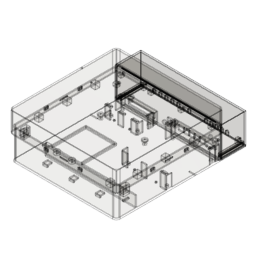
completed (Autodesk Fusion 360 design; units mm, degrees)
part number: 2026-08-16-23-06-11-456
Autodesk Fusion 360 part; units mm, degrees
(part 1 of 2)
sketch "Sketch1" plane through (0, 0, 0) normal (0, 0, 1) x (1, 0, 0)
  line L0 (140, 137) -> (-140, 137)
  line L1 (-140, 137) -> (-140, -140)
  line L2 (-140, -140) -> (140, -140)
  line L3 (140, -140) -> (140, 137)
extrude "Extrude1" add sketch "Sketch1" along normal blind 3 makes body 1
sketch "Sketch2" plane through (0, 0, 0) normal (0, 0, 1) x (1, 0, 0)
  line L0 (-137, 137) -> (-140, 137)
  line L1 (-140, 137) -> (-140, -140)
  line L2 (-140, -140) -> (-137, -140)
  line L3 (-137, -140) -> (-137, 137)
extrude "Extrude2" add sketch "Sketch2" along normal blind 77 from surface at 3 bodies 1
sketch "Sketch3" plane through (0, 0, 0) normal (0, 0, 1) x (1, 0, 0)
  line L0 (140, 137) -> (137, 137)
  line L1 (137, 137) -> (137, -140)
  line L2 (137, -140) -> (140, -140)
  line L3 (140, -140) -> (140, 137)
extrude "Extrude3" add sketch "Sketch3" along normal blind 77 from surface at 3 bodies 1
sketch "Sketch4" plane through (0, 0, 0) normal (0, 0, 1) x (1, 0, 0)
  line L0 (140, -137) -> (-140, -137)
  line L1 (-140, -137) -> (-140, -140)
  line L2 (-140, -140) -> (140, -140)
  line L3 (140, -140) -> (140, -137)
extrude "Extrude4" add sketch "Sketch4" along normal blind 77 from surface at 3 bodies 1
sketch "Sketch5" plane through (0, 0, 0) normal (0, 0, 1) x (1, 0, 0)
  line L0 (137, 137) -> (-137, 137)
  line L1 (-137, 137) -> (-137, 134)
  line L2 (-137, 134) -> (137, 134)
  line L3 (137, 134) -> (137, 137)
extrude "Extrude5" add sketch "Sketch5" along normal blind 8 from surface at 72 bodies 1
fillet "Fillet1" radius 7 2 edges at (-137, -137, 41.5) (137, -137, 41.5) on bodies 1
fillet "Fillet2" radius 10 2 edges at (-140, -140, 40) (140, -140, 40) on bodies 1
sketch "Sketch6" plane through (0, 0, 0) normal (0, 0, 1) x (1, 0, 0)
  circle A0 centre (27, 122.5) radius 3.5
extrude "Extrude6" add sketch "Sketch6" along normal blind 3.5 from surface at 3 bodies 1
sketch "Sketch7" plane through (0, 0, 0) normal (0, 0, 1) x (1, 0, 0)
  circle A0 centre (27, 5.5) radius 3.5
extrude "Extrude7" add sketch "Sketch7" along normal blind 3.5 from surface at 3 bodies 1
sketch "Sketch8" plane through (0, 0, 0) normal (0, 0, 1) x (1, 0, 0)
  circle A0 centre (129, 122.5) radius 3.5
extrude "Extrude8" add sketch "Sketch8" along normal blind 3.5 from surface at 3 bodies 1
sketch "Sketch9" plane through (0, 0, 0) normal (0, 0, 1) x (1, 0, 0)
  circle A0 centre (129, 5.5) radius 3.5
extrude "Extrude9" add sketch "Sketch9" along normal blind 3.5 from surface at 3 bodies 1
sketch "Sketch10" plane through (0, 0, 0) normal (0, 0, 1) x (1, 0, 0)
  line L0 (34.5, -3) -> (20.5, -3)
  line L1 (20.5, -3) -> (20.5, -5.5)
  line L2 (20.5, -5.5) -> (34.5, -5.5)
  line L3 (34.5, -5.5) -> (34.5, -3)
extrude "Extrude10" add sketch "Sketch10" along normal blind 32.6 from surface at 3 bodies 1
sketch "Sketch11" plane through (0, 0, 0) normal (0, 0, 1) x (1, 0, 0)
  line L0 (85, -3) -> (71, -3)
  line L1 (71, -3) -> (71, -5.5)
  line L2 (71, -5.5) -> (85, -5.5)
  line L3 (85, -5.5) -> (85, -3)
extrude "Extrude11" add sketch "Sketch11" along normal blind 32.6 from surface at 3 bodies 1
sketch "Sketch12" plane through (0, 0, 0) normal (0, 0, 1) x (1, 0, 0)
  line L0 (135.5, -3) -> (121.5, -3)
  line L1 (121.5, -3) -> (121.5, -5.5)
  line L2 (121.5, -5.5) -> (135.5, -5.5)
  line L3 (135.5, -5.5) -> (135.5, -3)
extrude "Extrude12" add sketch "Sketch12" along normal blind 36.5 from surface at 3 bodies 1
sketch "Sketch13" plane through (0, 0, 0) normal (0, 0, 1) x (1, 0, 0)
  line L0 (135.5, 2.25) -> (121.5, 2.25)
  line L1 (121.5, 2.25) -> (121.5, -4.25)
  line L2 (121.5, -4.25) -> (135.5, -4.25)
  line L3 (135.5, -4.25) -> (135.5, 2.25)
extrude "Extrude13" add sketch "Sketch13" along normal blind 3 from surface at 35.5 bodies 1
sketch "Sketch14" plane through (0, 0, 0) normal (0, 0, 1) x (1, 0, 0)
  line L0 (20.5, 11) -> (18, 11)
  line L1 (18, 11) -> (18, -3)
  line L2 (18, -3) -> (20.5, -3)
  line L3 (20.5, -3) -> (20.5, 11)
extrude "Extrude14" add sketch "Sketch14" along normal blind 32.5 from surface at 3 bodies 1
sketch "Sketch15" plane through (0, 0, 0) normal (0, 0, 1) x (1, 0, 0)
  line L0 (20.5, 126) -> (18, 126)
  line L1 (18, 126) -> (18, 112)
  line L2 (18, 112) -> (20.5, 112)
  line L3 (20.5, 112) -> (20.5, 126)
extrude "Extrude15" add sketch "Sketch15" along normal blind 37.5 from surface at 3 bodies 1
sketch "Sketch16" plane through (0, 0, 0) normal (0, 0, 1) x (1, 0, 0)
  line L0 (24.5, 126) -> (18, 126)
  line L1 (18, 126) -> (18, 112)
  line L2 (18, 112) -> (24.5, 112)
  line L3 (24.5, 112) -> (24.5, 126)
extrude "Extrude16" add sketch "Sketch16" along normal blind 3 from surface at 35.5 bodies 1
sketch "Sketch17" plane through (0, 0, 0) normal (0, 0, 1) x (1, 0, 0)
  line L0 (51, 0.5) -> (48, 0.5)
  line L1 (48, 0.5) -> (48, -2.5)
  line L2 (48, -2.5) -> (51, -2.5)
  line L3 (51, -2.5) -> (51, 0.5)
extrude "Extrude17" add sketch "Sketch17" along normal blind 3 from surface at 3 bodies 1
sketch "Sketch18" plane through (0, 0, 0) normal (0, 0, 1) x (1, 0, 0)
  line L0 (138, 11) -> (135.5, 11)
  line L1 (135.5, 11) -> (135.5, -3)
  line L2 (135.5, -3) -> (138, -3)
  line L3 (138, -3) -> (138, 11)
extrude "Extrude18" add sketch "Sketch18" along normal blind 32.5 from surface at 3 bodies 1
sketch "Sketch19" plane through (0, 0, 0) normal (0, 0, 1) x (1, 0, 0)
  line L0 (138, 126) -> (135.5, 126)
  line L1 (135.5, 126) -> (135.5, 112)
  line L2 (135.5, 112) -> (138, 112)
  line L3 (138, 112) -> (138, 126)
extrude "Extrude19" add sketch "Sketch19" along normal blind 37.5 from surface at 3 bodies 1
sketch "Sketch20" plane through (0, 0, 0) normal (0, 0, 1) x (1, 0, 0)
  line L0 (138, 126) -> (131.5, 126)
  line L1 (131.5, 126) -> (131.5, 112)
  line L2 (131.5, 112) -> (138, 112)
  line L3 (138, 112) -> (138, 126)
extrude "Extrude20" add sketch "Sketch20" along normal blind 3 from surface at 35.5 bodies 1
sketch "Sketch21" plane through (0, 0, 0) normal (0, 0, 1) x (1, 0, 0)
  line L0 (108, 0.5) -> (105, 0.5)
  line L1 (105, 0.5) -> (105, -2.5)
  line L2 (105, -2.5) -> (108, -2.5)
  line L3 (108, -2.5) -> (108, 0.5)
extrude "Extrude21" add sketch "Sketch21" along normal blind 3 from surface at 3 bodies 1
sketch "Sketch22" plane through (0, 0, 0) normal (0, 0, 1) x (1, 0, 0)
  circle A0 centre (-106, 122.5) radius 3.5
extrude "Extrude22" add sketch "Sketch22" along normal blind 3.5 from surface at 3 bodies 1
sketch "Sketch23" plane through (0, 0, 0) normal (0, 0, 1) x (1, 0, 0)
  circle A0 centre (-106, 92.5) radius 3.5
extrude "Extrude23" add sketch "Sketch23" along normal blind 3.5 from surface at 3 bodies 1
sketch "Sketch24" plane through (0, 0, 0) normal (0, 0, 1) x (1, 0, 0)
  circle A0 centre (-36, 122.5) radius 3.5
extrude "Extrude24" add sketch "Sketch24" along normal blind 3.5 from surface at 3 bodies 1
sketch "Sketch25" plane through (0, 0, 0) normal (0, 0, 1) x (1, 0, 0)
  circle A0 centre (-36, 92.5) radius 3.5
extrude "Extrude25" add sketch "Sketch25" along normal blind 3.5 from surface at 3 bodies 1
sketch "Sketch26" plane through (0, 0, 0) normal (0, 0, 1) x (1, 0, 0)
  line L0 (-98.5, 84) -> (-112.5, 84)
  line L1 (-112.5, 84) -> (-112.5, 81.5)
  line L2 (-112.5, 81.5) -> (-98.5, 81.5)
  line L3 (-98.5, 81.5) -> (-98.5, 84)
extrude "Extrude26" add sketch "Sketch26" along normal blind 30.5 from surface at 3 bodies 1
sketch "Sketch27" plane through (0, 0, 0) normal (0, 0, 1) x (1, 0, 0)
  line L0 (-98.5, 89.25) -> (-112.5, 89.25)
  line L1 (-112.5, 89.25) -> (-112.5, 82.75)
  line L2 (-112.5, 82.75) -> (-98.5, 82.75)
  line L3 (-98.5, 82.75) -> (-98.5, 89.25)
extrude "Extrude27" add sketch "Sketch27" along normal blind 3 from surface at 29.5 bodies 1
sketch "Sketch28" plane through (0, 0, 0) normal (0, 0, 1) x (1, 0, 0)
  line L0 (-64, 84) -> (-78, 84)
  line L1 (-78, 84) -> (-78, 81.5)
  line L2 (-78, 81.5) -> (-64, 81.5)
  line L3 (-64, 81.5) -> (-64, 84)
extrude "Extrude28" add sketch "Sketch28" along normal blind 30.5 from surface at 3 bodies 1
sketch "Sketch29" plane through (0, 0, 0) normal (0, 0, 1) x (1, 0, 0)
  line L0 (-64, 89.25) -> (-78, 89.25)
  line L1 (-78, 89.25) -> (-78, 82.75)
  line L2 (-78, 82.75) -> (-64, 82.75)
  line L3 (-64, 82.75) -> (-64, 89.25)
extrude "Extrude29" add sketch "Sketch29" along normal blind 3 from surface at 29.5 bodies 1
sketch "Sketch30" plane through (0, 0, 0) normal (0, 0, 1) x (1, 0, 0)
  line L0 (-29.5, 84) -> (-43.5, 84)
  line L1 (-43.5, 84) -> (-43.5, 81.5)
  line L2 (-43.5, 81.5) -> (-29.5, 81.5)
  line L3 (-29.5, 81.5) -> (-29.5, 84)
extrude "Extrude30" add sketch "Sketch30" along normal blind 30.5 from surface at 3 bodies 1
sketch "Sketch31" plane through (0, 0, 0) normal (0, 0, 1) x (1, 0, 0)
  line L0 (-29.5, 89.25) -> (-43.5, 89.25)
  line L1 (-43.5, 89.25) -> (-43.5, 82.75)
  line L2 (-43.5, 82.75) -> (-29.5, 82.75)
  line L3 (-29.5, 82.75) -> (-29.5, 89.25)
extrude "Extrude31" add sketch "Sketch31" along normal blind 3 from surface at 29.5 bodies 1
sketch "Sketch32" plane through (0, 0, 0) normal (0, 0, 1) x (1, 0, 0)
  line L0 (-112.5, 98) -> (-115, 98)
  line L1 (-115, 98) -> (-115, 84)
  line L2 (-115, 84) -> (-112.5, 84)
  line L3 (-112.5, 84) -> (-112.5, 98)
extrude "Extrude32" add sketch "Sketch32" along normal blind 8 from surface at 3 bodies 1
sketch "Sketch33" plane through (0, 0, 0) normal (0, 0, 1) x (1, 0, 0)
  line L0 (-112.5, 126) -> (-115, 126)
  line L1 (-115, 126) -> (-115, 112)
  line L2 (-115, 112) -> (-112.5, 112)
  line L3 (-112.5, 112) -> (-112.5, 126)
extrude "Extrude33" add sketch "Sketch33" along normal blind 31.5 from surface at 3 bodies 1
sketch "Sketch34" plane through (0, 0, 0) normal (0, 0, 1) x (1, 0, 0)
  line L0 (-108.5, 126) -> (-115, 126)
  line L1 (-115, 126) -> (-115, 112)
  line L2 (-115, 112) -> (-108.5, 112)
  line L3 (-108.5, 112) -> (-108.5, 126)
extrude "Extrude34" add sketch "Sketch34" along normal blind 3 from surface at 29.5 bodies 1
sketch "Sketch35" plane through (0, 0, 0) normal (0, 0, 1) x (1, 0, 0)
  line L0 (-90, 87.5) -> (-93, 87.5)
  line L1 (-93, 87.5) -> (-93, 84.5)
  line L2 (-93, 84.5) -> (-90, 84.5)
  line L3 (-90, 84.5) -> (-90, 87.5)
extrude "Extrude35" add sketch "Sketch35" along normal blind 3 from surface at 3 bodies 1
sketch "Sketch36" plane through (0, 0, 0) normal (0, 0, 1) x (1, 0, 0)
  line L0 (-27, 98) -> (-29.5, 98)
  line L1 (-29.5, 98) -> (-29.5, 84)
  line L2 (-29.5, 84) -> (-27, 84)
  line L3 (-27, 84) -> (-27, 98)
extrude "Extrude36" add sketch "Sketch36" along normal blind 26.5 from surface at 3 bodies 1
sketch "Sketch37" plane through (0, 0, 0) normal (0, 0, 1) x (1, 0, 0)
  line L0 (-27, 126) -> (-29.5, 126)
  line L1 (-29.5, 126) -> (-29.5, 112)
  line L2 (-29.5, 112) -> (-27, 112)
  line L3 (-27, 112) -> (-27, 126)
extrude "Extrude37" add sketch "Sketch37" along normal blind 31.5 from surface at 3 bodies 1
sketch "Sketch38" plane through (0, 0, 0) normal (0, 0, 1) x (1, 0, 0)
  line L0 (-27, 126) -> (-33.5, 126)
  line L1 (-33.5, 126) -> (-33.5, 112)
  line L2 (-33.5, 112) -> (-27, 112)
  line L3 (-27, 112) -> (-27, 126)
extrude "Extrude38" add sketch "Sketch38" along normal blind 3 from surface at 29.5 bodies 1
sketch "Sketch39" plane through (0, 0, 0) normal (0, 0, 1) x (1, 0, 0)
  line L0 (-49, 87.5) -> (-52, 87.5)
  line L1 (-52, 87.5) -> (-52, 84.5)
  line L2 (-52, 84.5) -> (-49, 84.5)
  line L3 (-49, 84.5) -> (-49, 87.5)
extrude "Extrude39" add sketch "Sketch39" along normal blind 3 from surface at 3 bodies 1
sketch "Sketch40" plane through (0, 0, 0) normal (0, 0, 1) x (1, 0, 0)
  line L0 (-32.2, 32.8) -> (-113.8, 32.8)
  line L1 (-113.8, 32.8) -> (-113.8, 30.3)
  line L2 (-113.8, 30.3) -> (-32.2, 30.3)
  line L3 (-32.2, 30.3) -> (-32.2, 32.8)
extrude "Extrude40" add sketch "Sketch40" along normal blind 5.5 from surface at 3 bodies 1
sketch "Sketch41" plane through (0, 0, 0) normal (0, 0, 1) x (1, 0, 0)
  line L0 (-111.3, 30.3) -> (-113.8, 30.3)
  line L1 (-113.8, 30.3) -> (-113.8, -58.3)
  line L2 (-113.8, -58.3) -> (-111.3, -58.3)
  line L3 (-111.3, -58.3) -> (-111.3, 30.3)
extrude "Extrude41" add sketch "Sketch41" along normal blind 5.5 from surface at 3 bodies 1
sketch "Sketch42" plane through (0, 0, 0) normal (0, 0, 1) x (1, 0, 0)
  line L0 (-32.2, 30.3) -> (-34.7, 30.3)
  line L1 (-34.7, 30.3) -> (-34.7, -58.3)
  line L2 (-34.7, -58.3) -> (-32.2, -58.3)
  line L3 (-32.2, -58.3) -> (-32.2, 30.3)
extrude "Extrude42" add sketch "Sketch42" along normal blind 5.5 from surface at 3 bodies 1
sketch "Sketch43" plane through (0, 0, 0) normal (0, 0, 1) x (1, 0, 0)
  circle A0 centre (-93, -65) radius 7
extrude "Extrude43" add sketch "Sketch43" along normal blind 6 from surface at 3 bodies 1
sketch "Sketch44" plane through (0, 0, 0) normal (0, 0, 1) x (1, 0, 0)
  circle A0 centre (-93, -65) radius 1.7
extrude "Extrude44" cut sketch "Sketch44" along normal blind 7 from surface at 2 bodies 1
sketch "Sketch45" plane through (0, 0, 0) normal (0, 0, 1) x (1, 0, 0)
  circle A0 centre (-53, -65) radius 7
extrude "Extrude45" add sketch "Sketch45" along normal blind 6 from surface at 3 bodies 1
sketch "Sketch46" plane through (0, 0, 0) normal (0, 0, 1) x (1, 0, 0)
  circle A0 centre (-53, -65) radius 1.7
extrude "Extrude46" cut sketch "Sketch46" along normal blind 7 from surface at 2 bodies 1
sketch "Sketch47" plane through (0, 0, 0) normal (0, 0, 1) x (1, 0, 0)
  line L0 (137, -83.5) -> (-103, -83.5)
  line L1 (-103, -83.5) -> (-103, -86.5)
  line L2 (-103, -86.5) -> (137, -86.5)
  line L3 (137, -86.5) -> (137, -83.5)
extrude "Extrude47" add sketch "Sketch47" along normal blind 29 from surface at 3 bodies 1
sketch "Sketch48" plane through (0, 0, 0) normal (0, 0, 1) x (1, 0, 0)
  line L0 (-47, -133.5) -> (-59, -133.5)
  line L1 (-59, -133.5) -> (-59, -138.5)
  line L2 (-59, -138.5) -> (-47, -138.5)
  line L3 (-47, -138.5) -> (-47, -133.5)
extrude "Extrude48" add sketch "Sketch48" along normal blind 6 from surface at 29 bodies 1
sketch "Sketch49" plane through (0, 0, 0) normal (0, 0, 1) x (1, 0, 0)
  line L0 (-47, -123.5) -> (-59, -123.5)
  line L1 (-59, -123.5) -> (-59, -135.5)
  line L2 (-59, -135.5) -> (-47, -135.5)
  line L3 (-47, -135.5) -> (-47, -123.5)
extrude "Extrude49" add sketch "Sketch49" along normal blind 3 from surface at 32 bodies 1
sketch "Sketch50" plane through (0, 0, 0) normal (0, 0, 1) x (1, 0, 0)
  line L0 (23, -133.5) -> (11, -133.5)
  line L1 (11, -133.5) -> (11, -138.5)
  line L2 (11, -138.5) -> (23, -138.5)
  line L3 (23, -138.5) -> (23, -133.5)
extrude "Extrude50" add sketch "Sketch50" along normal blind 6 from surface at 29 bodies 1
sketch "Sketch51" plane through (0, 0, 0) normal (0, 0, 1) x (1, 0, 0)
  line L0 (23, -123.5) -> (11, -123.5)
  line L1 (11, -123.5) -> (11, -135.5)
  line L2 (11, -135.5) -> (23, -135.5)
  line L3 (23, -135.5) -> (23, -123.5)
extrude "Extrude51" add sketch "Sketch51" along normal blind 3 from surface at 32 bodies 1
sketch "Sketch52" plane through (0, 0, 0) normal (0, 0, 1) x (1, 0, 0)
  line L0 (93, -133.5) -> (81, -133.5)
  line L1 (81, -133.5) -> (81, -138.5)
  line L2 (81, -138.5) -> (93, -138.5)
  line L3 (93, -138.5) -> (93, -133.5)
extrude "Extrude52" add sketch "Sketch52" along normal blind 6 from surface at 29 bodies 1
sketch "Sketch53" plane through (0, 0, 0) normal (0, 0, 1) x (1, 0, 0)
  line L0 (93, -123.5) -> (81, -123.5)
  line L1 (81, -123.5) -> (81, -135.5)
  line L2 (81, -135.5) -> (93, -135.5)
  line L3 (93, -135.5) -> (93, -123.5)
extrude "Extrude53" add sketch "Sketch53" along normal blind 3 from surface at 32 bodies 1
sketch "Sketch54" plane through (0, 0, 0) normal (0, 0, 1) x (1, 0, 0)
  line L0 (139, -102.5) -> (133, -102.5)
  line L1 (133, -102.5) -> (133, -117.5)
  line L2 (133, -117.5) -> (139, -117.5)
  line L3 (139, -117.5) -> (139, -102.5)
extrude "Extrude54" add sketch "Sketch54" along normal blind 3 from surface at 32 bodies 1
sketch "Sketch55" plane through (0, 0, 0) normal (0, 0, 1) x (1, 0, 0)
  line L0 (-89, -83.5) -> (-101, -83.5)
  line L1 (-101, -83.5) -> (-101, -86.5)
  line L2 (-101, -86.5) -> (-89, -86.5)
  line L3 (-89, -86.5) -> (-89, -83.5)
extrude "Extrude55" add sketch "Sketch55" along normal blind 6 from surface at 29 bodies 1
sketch "Sketch56" plane through (0, 0, 0) normal (0, 0, 1) x (1, 0, 0)
  line L0 (-89, -84.5) -> (-101, -84.5)
  line L1 (-101, -84.5) -> (-101, -96.5)
  line L2 (-101, -96.5) -> (-89, -96.5)
  line L3 (-89, -96.5) -> (-89, -84.5)
extrude "Extrude56" add sketch "Sketch56" along normal blind 3 from surface at 32 bodies 1
sketch "Sketch57" plane through (0, 0, 0) normal (0, 0, 1) x (1, 0, 0)
  line L0 (139, -102) -> (127, -102)
  line L1 (127, -102) -> (127, -118)
  line L2 (127, -118) -> (139, -118)
  line L3 (139, -118) -> (139, -102)
extrude "Extrude57" add sketch "Sketch57" along normal blind 22 from surface at 44 bodies 1
sketch "Sketch58" plane through (0, 0, 0) normal (0, 0, 1) x (1, 0, 0)
  line L0 (136.5, -99) -> (129.5, -99)
  line L1 (129.5, -99) -> (129.5, -121)
  line L2 (129.5, -121) -> (136.5, -121)
  line L3 (136.5, -121) -> (136.5, -99)
extrude "Extrude58" cut sketch "Sketch58" along normal blind 12 from surface at 49 bodies 1
sketch "Sketch59" plane through (0, 0, 0) normal (0, 0, 1) x (1, 0, 0)
  line L0 (-127, -102) -> (-139, -102)
  line L1 (-139, -102) -> (-139, -118)
  line L2 (-139, -118) -> (-127, -118)
  line L3 (-127, -118) -> (-127, -102)
extrude "Extrude59" add sketch "Sketch59" along normal blind 22 from surface at 44 bodies 1
sketch "Sketch60" plane through (0, 0, 0) normal (0, 0, 1) x (1, 0, 0)
  line L0 (-129.5, -99) -> (-136.5, -99)
  line L1 (-136.5, -99) -> (-136.5, -121)
  line L2 (-136.5, -121) -> (-129.5, -121)
  line L3 (-129.5, -121) -> (-129.5, -99)
extrude "Extrude60" cut sketch "Sketch60" along normal blind 12 from surface at 49 bodies 1
sketch "Sketch61" plane through (0, 0, 0) normal (0, 1, 0) x (1, 0, 0)
  circle A0 centre (-60, 56) radius 5.5
extrude "Extrude61" cut sketch "Sketch61" along normal mid plane 5 from surface at -139 bodies 1
sketch "Sketch62" plane through (0, 0, 0) normal (0, 1, 0) x (1, 0, 0)
  line L0 (-57.5, 56) -> (-62.5, 56)
  line L1 (-62.5, 56) -> (-62.5, 38)
  line L2 (-62.5, 38) -> (-57.5, 38)
  line L3 (-57.5, 38) -> (-57.5, 56)
extrude "Extrude62" cut sketch "Sketch62" along normal mid plane 5 from surface at -139 bodies 1
sketch "Sketch63" plane through (0, 0, 0) normal (0, 1, 0) x (1, 0, 0)
  circle A0 centre (60, 56) radius 5.5
extrude "Extrude63" cut sketch "Sketch63" along normal mid plane 5 from surface at -139 bodies 1
sketch "Sketch64" plane through (0, 0, 0) normal (0, 1, 0) x (1, 0, 0)
  line L0 (62.5, 56) -> (57.5, 56)
  line L1 (57.5, 56) -> (57.5, 38)
  line L2 (57.5, 38) -> (62.5, 38)
  line L3 (62.5, 38) -> (62.5, 56)
extrude "Extrude64" cut sketch "Sketch64" along normal mid plane 5 from surface at -139 bodies 1
sketch "Sketch65" plane through (0, 0, 0) normal (0, 0, 1) x (1, 0, 0)
  line L0 (-125, -69) -> (-137, -69)
  line L1 (-137, -69) -> (-137, -81)
  line L2 (-137, -81) -> (-125, -81)
  line L3 (-125, -81) -> (-125, -69)
extrude "Extrude65" add sketch "Sketch65" along normal blind 12 from surface at 66 bodies 1
sketch "Sketch66" plane through (0, 0, 0) normal (1, 0, 0) x (0, 0, -1)
  circle A0 centre (-75, 72) radius 1.3
extrude "Extrude66" cut sketch "Sketch66" along normal mid plane 30 from surface at -137 bodies 1
sketch "Sketch67" plane through (0, 0, 0) normal (0, 0, 1) x (1, 0, 0)
  line L0 (-125, 6) -> (-137, 6)
  line L1 (-137, 6) -> (-137, -6)
  line L2 (-137, -6) -> (-125, -6)
  line L3 (-125, -6) -> (-125, 6)
extrude "Extrude67" add sketch "Sketch67" along normal blind 12 from surface at 66 bodies 1
sketch "Sketch68" plane through (0, 0, 0) normal (1, 0, 0) x (0, 0, -1)
  circle A0 centre (0, 72) radius 1.3
extrude "Extrude68" cut sketch "Sketch68" along normal mid plane 30 from surface at -137 bodies 1
sketch "Sketch69" plane through (0, 0, 0) normal (0, 0, 1) x (1, 0, 0)
  line L0 (-125, 81) -> (-137, 81)
  line L1 (-137, 81) -> (-137, 69)
  line L2 (-137, 69) -> (-125, 69)
  line L3 (-125, 69) -> (-125, 81)
extrude "Extrude69" add sketch "Sketch69" along normal blind 12 from surface at 66 bodies 1
sketch "Sketch70" plane through (0, 0, 0) normal (1, 0, 0) x (0, 0, -1)
  circle A0 centre (75, 72) radius 1.3
extrude "Extrude70" cut sketch "Sketch70" along normal mid plane 30 from surface at -137 bodies 1
sketch "Sketch71" plane through (0, 0, 0) normal (0, 0, 1) x (1, 0, 0)
  line L0 (137, -69) -> (125, -69)
  line L1 (125, -69) -> (125, -81)
  line L2 (125, -81) -> (137, -81)
  line L3 (137, -81) -> (137, -69)
extrude "Extrude71" add sketch "Sketch71" along normal blind 12 from surface at 66 bodies 1
sketch "Sketch72" plane through (0, 0, 0) normal (1, 0, 0) x (0, 0, -1)
  circle A0 centre (-75, 72) radius 1.3
extrude "Extrude72" cut sketch "Sketch72" along normal mid plane 30 from surface at 137 bodies 1
sketch "Sketch73" plane through (0, 0, 0) normal (0, 0, 1) x (1, 0, 0)
  line L0 (137, 6) -> (125, 6)
  line L1 (125, 6) -> (125, -6)
  line L2 (125, -6) -> (137, -6)
  line L3 (137, -6) -> (137, 6)
extrude "Extrude73" add sketch "Sketch73" along normal blind 12 from surface at 66 bodies 1
sketch "Sketch74" plane through (0, 0, 0) normal (1, 0, 0) x (0, 0, -1)
  circle A0 centre (0, 72) radius 1.3
extrude "Extrude74" cut sketch "Sketch74" along normal mid plane 30 from surface at 137 bodies 1
sketch "Sketch75" plane through (0, 0, 0) normal (0, 0, 1) x (1, 0, 0)
  line L0 (137, 81) -> (125, 81)
  line L1 (125, 81) -> (125, 69)
  line L2 (125, 69) -> (137, 69)
  line L3 (137, 69) -> (137, 81)
extrude "Extrude75" add sketch "Sketch75" along normal blind 12 from surface at 66 bodies 1
sketch "Sketch76" plane through (0, 0, 0) normal (1, 0, 0) x (0, 0, -1)
  circle A0 centre (75, 72) radius 1.3
extrude "Extrude76" cut sketch "Sketch76" along normal mid plane 30 from surface at 137 bodies 1
sketch "Sketch77" plane through (0, 0, 0) normal (0, 0, 1) x (1, 0, 0)
  line L0 (-109, -125) -> (-121, -125)
  line L1 (-121, -125) -> (-121, -137)
  line L2 (-121, -137) -> (-109, -137)
  line L3 (-109, -137) -> (-109, -125)
extrude "Extrude77" add sketch "Sketch77" along normal blind 12 from surface at 66 bodies 1
sketch "Sketch78" plane through (0, 0, 0) normal (0, 1, 0) x (1, 0, 0)
  circle A0 centre (-115, 72) radius 1.3
extrude "Extrude78" cut sketch "Sketch78" along normal mid plane 30 from surface at -137 bodies 1
sketch "Sketch79" plane through (0, 0, 0) normal (0, 0, 1) x (1, 0, 0)
  line L0 (121, -125) -> (109, -125)
  line L1 (109, -125) -> (109, -137)
  line L2 (109, -137) -> (121, -137)
  line L3 (121, -137) -> (121, -125)
extrude "Extrude79" add sketch "Sketch79" along normal blind 12 from surface at 66 bodies 1
sketch "Sketch80" plane through (0, 0, 0) normal (0, 1, 0) x (1, 0, 0)
  circle A0 centre (115, 72) radius 1.3
extrude "Extrude80" cut sketch "Sketch80" along normal mid plane 30 from surface at -137 bodies 1
sketch "Sketch81" plane through (0, 0, 0) normal (0, 0, 1) x (1, 0, 0)
  line L0 (-140, -41) -> (-141.2, -41)
  line L1 (-141.2, -41) -> (-141.2, -49)
  line L2 (-141.2, -49) -> (-140, -49)
  line L3 (-140, -49) -> (-140, -41)
extrude "Extrude81" add sketch "Sketch81" along normal blind 2.5 from surface at 71 bodies 1
sketch "Sketch82" plane through (0, 0, 0) normal (0, 0, 1) x (1, 0, 0)
  line L0 (-140, -41) -> (-140.6, -41)
  line L1 (-140.6, -41) -> (-140.6, -49)
  line L2 (-140.6, -49) -> (-140, -49)
  line L3 (-140, -49) -> (-140, -41)
extrude "Extrude82" add sketch "Sketch82" along normal blind 2.5 from surface at 73.5 bodies 1
sketch "Sketch83" plane through (0, 0, 0) normal (0, 0, 1) x (1, 0, 0)
  line L0 (141.2, -41) -> (140, -41)
  line L1 (140, -41) -> (140, -49)
  line L2 (140, -49) -> (141.2, -49)
  line L3 (141.2, -49) -> (141.2, -41)
extrude "Extrude83" add sketch "Sketch83" along normal blind 2.5 from surface at 71 bodies 1
sketch "Sketch84" plane through (0, 0, 0) normal (0, 0, 1) x (1, 0, 0)
  line L0 (140.6, -41) -> (140, -41)
  line L1 (140, -41) -> (140, -49)
  line L2 (140, -49) -> (140.6, -49)
  line L3 (140.6, -49) -> (140.6, -41)
extrude "Extrude84" add sketch "Sketch84" along normal blind 2.5 from surface at 73.5 bodies 1
sketch "Sketch85" plane through (0, 0, 0) normal (0, 0, 1) x (1, 0, 0)
  line L0 (-140, 49) -> (-141.2, 49)
  line L1 (-141.2, 49) -> (-141.2, 41)
  line L2 (-141.2, 41) -> (-140, 41)
  line L3 (-140, 41) -> (-140, 49)
extrude "Extrude85" add sketch "Sketch85" along normal blind 2.5 from surface at 71 bodies 1
sketch "Sketch86" plane through (0, 0, 0) normal (0, 0, 1) x (1, 0, 0)
  line L0 (-140, 49) -> (-140.6, 49)
  line L1 (-140.6, 49) -> (-140.6, 41)
  line L2 (-140.6, 41) -> (-140, 41)
  line L3 (-140, 41) -> (-140, 49)
extrude "Extrude86" add sketch "Sketch86" along normal blind 2.5 from surface at 73.5 bodies 1
sketch "Sketch87" plane through (0, 0, 0) normal (0, 0, 1) x (1, 0, 0)
  line L0 (141.2, 49) -> (140, 49)
  line L1 (140, 49) -> (140, 41)
  line L2 (140, 41) -> (141.2, 41)
  line L3 (141.2, 41) -> (141.2, 49)
extrude "Extrude87" add sketch "Sketch87" along normal blind 2.5 from surface at 71 bodies 1
sketch "Sketch88" plane through (0, 0, 0) normal (0, 0, 1) x (1, 0, 0)
  line L0 (140.6, 49) -> (140, 49)
  line L1 (140, 49) -> (140, 41)
  line L2 (140, 41) -> (140.6, 41)
  line L3 (140.6, 41) -> (140.6, 49)
extrude "Extrude88" add sketch "Sketch88" along normal blind 2.5 from surface at 73.5 bodies 1
sketch "Sketch89" plane through (0, 0, 0) normal (0, 0, 1) x (1, 0, 0)
  line L0 (-41, -140) -> (-49, -140)
  line L1 (-49, -140) -> (-49, -141.2)
  line L2 (-49, -141.2) -> (-41, -141.2)
  line L3 (-41, -141.2) -> (-41, -140)
extrude "Extrude89" add sketch "Sketch89" along normal blind 2.5 from surface at 71 bodies 1
sketch "Sketch90" plane through (0, 0, 0) normal (0, 0, 1) x (1, 0, 0)
  line L0 (-41, -140) -> (-49, -140)
  line L1 (-49, -140) -> (-49, -140.6)
  line L2 (-49, -140.6) -> (-41, -140.6)
  line L3 (-41, -140.6) -> (-41, -140)
extrude "Extrude90" add sketch "Sketch90" along normal blind 2.5 from surface at 73.5 bodies 1
sketch "Sketch91" plane through (0, 0, 0) normal (0, 0, 1) x (1, 0, 0)
  line L0 (49, -140) -> (41, -140)
  line L1 (41, -140) -> (41, -141.2)
  line L2 (41, -141.2) -> (49, -141.2)
  line L3 (49, -141.2) -> (49, -140)
extrude "Extrude91" add sketch "Sketch91" along normal blind 2.5 from surface at 71 bodies 1
sketch "Sketch92" plane through (0, 0, 0) normal (0, 0, 1) x (1, 0, 0)
  line L0 (49, -140) -> (41, -140)
  line L1 (41, -140) -> (41, -140.6)
  line L2 (41, -140.6) -> (49, -140.6)
  line L3 (49, -140.6) -> (49, -140)
extrude "Extrude92" add sketch "Sketch92" along normal blind 2.5 from surface at 73.5 bodies 1
sketch "Sketch93" plane through (0, 0, 0) normal (0, 0, 1) x (1, 0, 0)
  line L0 (-115.5, 137) -> (-124.5, 137)
  line L1 (-124.5, 137) -> (-124.5, 128)
  line L2 (-124.5, 128) -> (-115.5, 128)
  line L3 (-115.5, 128) -> (-115.5, 137)
extrude "Extrude93" add sketch "Sketch93" along normal blind 8 from surface at 68 bodies 1
sketch "Sketch94" plane through (0, 0, 0) normal (0, 1, 0) x (1, 0, 0)
  circle A0 centre (-120, 72) radius 1.3
extrude "Extrude94" cut sketch "Sketch94" along normal mid plane 16 from surface at 132.5 bodies 1
sketch "Sketch95" plane through (0, 0, 0) normal (0, 0, 1) x (1, 0, 0)
  line L0 (124.5, 137) -> (115.5, 137)
  line L1 (115.5, 137) -> (115.5, 128)
  line L2 (115.5, 128) -> (124.5, 128)
  line L3 (124.5, 128) -> (124.5, 137)
extrude "Extrude95" add sketch "Sketch95" along normal blind 8 from surface at 68 bodies 1
sketch "Sketch96" plane through (0, 0, 0) normal (0, 1, 0) x (1, 0, 0)
  circle A0 centre (120, 72) radius 1.3
extrude "Extrude96" cut sketch "Sketch96" along normal mid plane 16 from surface at 132.5 bodies 1
sketch "Sketch97" plane through (0, 0, 0) normal (0, 0, 1) x (1, 0, 0)
  line L0 (-35.5, 137) -> (-44.5, 137)
  line L1 (-44.5, 137) -> (-44.5, 128)
  line L2 (-44.5, 128) -> (-35.5, 128)
  line L3 (-35.5, 128) -> (-35.5, 137)
extrude "Extrude97" add sketch "Sketch97" along normal blind 8 from surface at 68 bodies 1
sketch "Sketch98" plane through (0, 0, 0) normal (0, 1, 0) x (1, 0, 0)
  circle A0 centre (-40, 72) radius 1.3
extrude "Extrude98" cut sketch "Sketch98" along normal mid plane 16 from surface at 132.5 bodies 1
sketch "Sketch99" plane through (0, 0, 0) normal (0, 0, 1) x (1, 0, 0)
  line L0 (44.5, 137) -> (35.5, 137)
  line L1 (35.5, 137) -> (35.5, 128)
  line L2 (35.5, 128) -> (44.5, 128)
  line L3 (44.5, 128) -> (44.5, 137)
extrude "Extrude99" add sketch "Sketch99" along normal blind 8 from surface at 68 bodies 1
sketch "Sketch100" plane through (0, 0, 0) normal (0, 1, 0) x (1, 0, 0)
  circle A0 centre (40, 72) radius 1.3
extrude "Extrude100" cut sketch "Sketch100" along normal mid plane 16 from surface at 132.5 bodies 1
sketch "Sketch101" plane through (0, 0, 0) normal (0, 0, 1) x (1, 0, 0)
  line L0 (-127, 137) -> (-137, 137)
  line L1 (-137, 137) -> (-137, 128)
  line L2 (-137, 128) -> (-127, 128)
  line L3 (-127, 128) -> (-127, 137)
extrude "Extrude101" add sketch "Sketch101" along normal blind 8 from surface at 40 bodies 1
sketch "Sketch102" plane through (0, 0, 0) normal (0, 1, 0) x (1, 0, 0)
  circle A0 centre (-132, 44) radius 1.3
extrude "Extrude102" cut sketch "Sketch102" along normal mid plane 16 from surface at 132.5 bodies 1
sketch "Sketch103" plane through (0, 0, 0) normal (0, 0, 1) x (1, 0, 0)
  line L0 (137, 137) -> (127, 137)
  line L1 (127, 137) -> (127, 128)
  line L2 (127, 128) -> (137, 128)
  line L3 (137, 128) -> (137, 137)
extrude "Extrude103" add sketch "Sketch103" along normal blind 8 from surface at 40 bodies 1
sketch "Sketch104" plane through (0, 0, 0) normal (0, 1, 0) x (1, 0, 0)
  circle A0 centre (132, 44) radius 1.3
extrude "Extrude104" cut sketch "Sketch104" along normal mid plane 16 from surface at 132.5 bodies 1
sketch "Sketch105" plane through (0, 0, 0) normal (0, 0, 1) x (1, 0, 0)
  line L0 (143, 143) -> (-143, 143)
  line L1 (-143, 143) -> (-143, -143)
  line L2 (-143, -143) -> (143, -143)
  line L3 (143, -143) -> (143, 143)
extrude "Extrude105" add sketch "Sketch105" along normal blind 3 separate body makes body 2
sketch "Sketch106" plane through (0, 0, 0) normal (0, 0, 1) x (1, 0, 0)
  line L0 (143, 143) -> (-143, 143)
  line L1 (-143, 143) -> (-143, -143)
  line L2 (-143, -143) -> (143, -143)
  line L3 (143, -143) -> (143, 143)
extrude "Extrude106" add sketch "Sketch106" along normal blind 52 from surface at 3 bodies 2
sketch "Sketch107" plane through (0, 0, 0) normal (0, 0, 1) x (1, 0, 0)
  line L0 (140.5, 140.5) -> (-140.5, 140.5)
  line L1 (-140.5, 140.5) -> (-140.5, -140.5)
  line L2 (-140.5, -140.5) -> (140.5, -140.5)
  line L3 (140.5, -140.5) -> (140.5, 140.5)
extrude "Extrude107" cut sketch "Sketch107" along normal blind 54 from surface at 3 bodies 2
fillet "Fillet3" radius 10 4 edges at (143, -143, 27.5) (-143, -143, 27.5) (-143, 143, 27.5) (143, 143, 27.5) on bodies 2
sketch "Sketch108" plane through (0, 0, 0) normal (0, 0, 1) x (1, 0, 0)
  circle A0 centre (11.5, -30) radius 6.5
extrude "Extrude108" add sketch "Sketch108" along normal blind 3 from surface at 3 bodies 2
sketch "Sketch109" plane through (0, 0, 0) normal (0, 0, 1) x (1, 0, 0)
  circle A0 centre (11.5, -30) radius 4.5
extrude "Extrude109" add sketch "Sketch109" along normal blind 10.8 from surface at 3 bodies 2
sketch "Sketch110" plane through (0, 0, 0) normal (0, 0, 1) x (1, 0, 0)
  circle A0 centre (11.5, -30) radius 1.3
extrude "Extrude110" cut sketch "Sketch110" along normal blind 11.8 from surface at 3 bodies 2
sketch "Sketch111" plane through (0, 0, 0) normal (0, 0, 1) x (1, 0, 0)
  circle A0 centre (-105.5, -30) radius 6.5
extrude "Extrude111" add sketch "Sketch111" along normal blind 3 from surface at 3 bodies 2
sketch "Sketch112" plane through (0, 0, 0) normal (0, 0, 1) x (1, 0, 0)
  circle A0 centre (-105.5, -30) radius 4.5
extrude "Extrude112" add sketch "Sketch112" along normal blind 10.8 from surface at 3 bodies 2
sketch "Sketch113" plane through (0, 0, 0) normal (0, 0, 1) x (1, 0, 0)
  circle A0 centre (-105.5, -30) radius 1.3
extrude "Extrude113" cut sketch "Sketch113" along normal blind 11.8 from surface at 3 bodies 2
sketch "Sketch114" plane through (0, 0, 0) normal (0, 0, 1) x (1, 0, 0)
  circle A0 centre (11.5, 50) radius 6.5
extrude "Extrude114" add sketch "Sketch114" along normal blind 3 from surface at 3 bodies 2
sketch "Sketch115" plane through (0, 0, 0) normal (0, 0, 1) x (1, 0, 0)
  circle A0 centre (11.5, 50) radius 4.5
extrude "Extrude115" add sketch "Sketch115" along normal blind 10.8 from surface at 3 bodies 2
sketch "Sketch116" plane through (0, 0, 0) normal (0, 0, 1) x (1, 0, 0)
  circle A0 centre (11.5, 50) radius 1.3
extrude "Extrude116" cut sketch "Sketch116" along normal blind 11.8 from surface at 3 bodies 2
sketch "Sketch117" plane through (0, 0, 0) normal (0, 0, 1) x (1, 0, 0)
  circle A0 centre (-105.5, 50) radius 6.5
extrude "Extrude117" add sketch "Sketch117" along normal blind 3 from surface at 3 bodies 2
sketch "Sketch118" plane through (0, 0, 0) normal (0, 0, 1) x (1, 0, 0)
  circle A0 centre (-105.5, 50) radius 4.5
extrude "Extrude118" add sketch "Sketch118" along normal blind 10.8 from surface at 3 bodies 2
sketch "Sketch119" plane through (0, 0, 0) normal (0, 0, 1) x (1, 0, 0)
  circle A0 centre (-105.5, 50) radius 1.3
extrude "Extrude119" cut sketch "Sketch119" along normal blind 11.8 from surface at 3 bodies 2
sketch "Sketch120" plane through (0, 0, 0) normal (0, 0, 1) x (1, 0, 0)
  line L0 (141.7, 10) -> (139.7, 10)
  line L1 (139.7, 10) -> (139.7, -10)
  line L2 (139.7, -10) -> (141.7, -10)
  line L3 (141.7, -10) -> (141.7, 10)
extrude "Extrude120" add sketch "Sketch120" along normal blind 2 from surface at 45 bodies 2
sketch "Sketch121" plane through (0, 0, 0) normal (0, 0, 1) x (1, 0, 0)
  line L0 (-139.7, 10) -> (-141.7, 10)
  line L1 (-141.7, 10) -> (-141.7, -10)
  line L2 (-141.7, -10) -> (-139.7, -10)
  line L3 (-139.7, -10) -> (-139.7, 10)
extrude "Extrude121" add sketch "Sketch121" along normal blind 2 from surface at 45 bodies 2
sketch "Sketch122" plane through (0, 0, 0) normal (0, 0, 1) x (1, 0, 0)
  line L0 (10, -139.7) -> (-10, -139.7)
  line L1 (-10, -139.7) -> (-10, -141.7)
  line L2 (-10, -141.7) -> (10, -141.7)
  line L3 (10, -141.7) -> (10, -139.7)
extrude "Extrude122" add sketch "Sketch122" along normal blind 2 from surface at 45 bodies 2
sketch "Sketch123" plane through (0, 0, 0) normal (0, 0, 1) x (1, 0, 0)
  line L0 (140.5, 144.5) -> (-140.5, 144.5)
  line L1 (-140.5, 144.5) -> (-140.5, 139)
  line L2 (-140.5, 139) -> (140.5, 139)
  line L3 (140.5, 139) -> (140.5, 144.5)
extrude "Extrude123" cut sketch "Sketch123" along normal blind 20 from surface at 36.5 bodies 2
sketch "Sketch124" plane through (0, 0, 0) normal (1, 0, 0) x (0, 0, -1)
  circle A0 centre (-75, 48) radius 1.7
extrude "Extrude124" cut sketch "Sketch124" along normal mid plane 6 from surface at -142 bodies 2
sketch "Sketch125" plane through (0, 0, 0) normal (1, 0, 0) x (0, 0, -1)
  circle A0 centre (0, 48) radius 1.7
extrude "Extrude125" cut sketch "Sketch125" along normal mid plane 6 from surface at -142 bodies 2
sketch "Sketch126" plane through (0, 0, 0) normal (1, 0, 0) x (0, 0, -1)
  circle A0 centre (75, 48) radius 1.7
extrude "Extrude126" cut sketch "Sketch126" along normal mid plane 6 from surface at -142 bodies 2
sketch "Sketch127" plane through (0, 0, 0) normal (1, 0, 0) x (0, 0, -1)
  circle A0 centre (-75, 48) radius 1.7
extrude "Extrude127" cut sketch "Sketch127" along normal mid plane 6 from surface at 142 bodies 2
sketch "Sketch128" plane through (0, 0, 0) normal (1, 0, 0) x (0, 0, -1)
  circle A0 centre (0, 48) radius 1.7
extrude "Extrude128" cut sketch "Sketch128" along normal mid plane 6 from surface at 142 bodies 2
sketch "Sketch129" plane through (0, 0, 0) normal (1, 0, 0) x (0, 0, -1)
  circle A0 centre (75, 48) radius 1.7
extrude "Extrude129" cut sketch "Sketch129" along normal mid plane 6 from surface at 142 bodies 2
sketch "Sketch130" plane through (0, 0, 0) normal (0, 1, 0) x (1, 0, 0)
  circle A0 centre (-115, 48) radius 1.7
extrude "Extrude130" cut sketch "Sketch130" along normal mid plane 6 from surface at -142 bodies 2
sketch "Sketch131" plane through (0, 0, 0) normal (0, 1, 0) x (1, 0, 0)
  circle A0 centre (115, 48) radius 1.7
extrude "Extrude131" cut sketch "Sketch131" along normal mid plane 6 from surface at -142 bodies 2
sketch "Sketch132" plane through (0, 0, 0) normal (0, 0, 1) x (1, 0, 0)
  line L0 (-139, -40) -> (-144, -40)
  line L1 (-144, -40) -> (-144, -50)
  line L2 (-144, -50) -> (-139, -50)
  line L3 (-139, -50) -> (-139, -40)
extrude "Extrude132" cut sketch "Sketch132" along normal blind 6.5 from surface at 43.5 bodies 2
sketch "Sketch133" plane through (0, 0, 0) normal (0, 0, 1) x (1, 0, 0)
  line L0 (144, -40) -> (139, -40)
  line L1 (139, -40) -> (139, -50)
  line L2 (139, -50) -> (144, -50)
  line L3 (144, -50) -> (144, -40)
extrude "Extrude133" cut sketch "Sketch133" along normal blind 6.5 from surface at 43.5 bodies 2
sketch "Sketch134" plane through (0, 0, 0) normal (0, 0, 1) x (1, 0, 0)
  line L0 (-139, 50) -> (-144, 50)
  line L1 (-144, 50) -> (-144, 40)
  line L2 (-144, 40) -> (-139, 40)
  line L3 (-139, 40) -> (-139, 50)
extrude "Extrude134" cut sketch "Sketch134" along normal blind 6.5 from surface at 43.5 bodies 2
sketch "Sketch135" plane through (0, 0, 0) normal (0, 0, 1) x (1, 0, 0)
  line L0 (144, 50) -> (139, 50)
  line L1 (139, 50) -> (139, 40)
  line L2 (139, 40) -> (144, 40)
  line L3 (144, 40) -> (144, 50)
extrude "Extrude135" cut sketch "Sketch135" along normal blind 6.5 from surface at 43.5 bodies 2
sketch "Sketch136" plane through (0, 0, 0) normal (0, 0, 1) x (1, 0, 0)
  line L0 (-40, -139) -> (-50, -139)
  line L1 (-50, -139) -> (-50, -144)
  line L2 (-50, -144) -> (-40, -144)
  line L3 (-40, -144) -> (-40, -139)
extrude "Extrude136" cut sketch "Sketch136" along normal blind 6.5 from surface at 43.5 bodies 2
sketch "Sketch137" plane through (0, 0, 0) normal (0, 0, 1) x (1, 0, 0)
  line L0 (50, -139) -> (40, -139)
  line L1 (40, -139) -> (40, -144)
  line L2 (40, -144) -> (50, -144)
  line L3 (50, -144) -> (50, -139)
extrude "Extrude137" cut sketch "Sketch137" along normal blind 6.5 from surface at 43.5 bodies 2
move_body "Move1" bodies 2 to x (-1, 0, 0) y (0, 1, 0) z (0, 0, -1) at (0, 0, 120)
sketch "Sketch138" plane through (0, 0, 0) normal (0, 0, 1) x (1, 0, 0)
  line L0 (140, 80) -> (-140, 80)
  line L1 (-140, 80) -> (-140, 0)
  line L2 (-140, 0) -> (140, 0)
  line L3 (140, 0) -> (140, 80)
extrude "Extrude138" add sketch "Sketch138" along normal blind 3 separate body makes body 3
fillet "Fillet4" radius 6 4 edges at (140, 0, 1.5) (-140, 0, 1.5) (-140, 80, 1.5) (140, 80, 1.5) on bodies 3
sketch "Sketch139" plane through (0, 0, 0) normal (0, 0, 1) x (1, 0, 0)
  circle A0 centre (-124, 21.5) radius 3.25
extrude "Extrude139" cut sketch "Sketch139" along normal blind 5 from surface at -1 bodies 3
sketch "Sketch140" plane through (0, 0, 0) normal (0, 0, 1) x (1, 0, 0)
  circle A0 centre (-116, 16.5) radius 1.25
extrude "Extrude140" cut sketch "Sketch140" along normal blind 5 from surface at -1 bodies 3
sketch "Sketch141" plane through (0, 0, 0) normal (0, 0, 1) x (1, 0, 0)
  line L0 (-108, 17.5) -> (-112, 17.5)
  line L1 (-112, 17.5) -> (-112, 14.5)
  line L2 (-112, 14.5) -> (-108, 14.5)
  line L3 (-108, 14.5) -> (-108, 17.5)
extrude "Extrude141" cut sketch "Sketch141" along normal blind 5 from surface at -1 bodies 3
sketch "Sketch142" plane through (0, 0, 0) normal (0, 0, 1) x (1, 0, 0)
  line L0 (-100, 17.5) -> (-104, 17.5)
  line L1 (-104, 17.5) -> (-104, 14.5)
  line L2 (-104, 14.5) -> (-100, 14.5)
  line L3 (-100, 14.5) -> (-100, 17.5)
extrude "Extrude142" cut sketch "Sketch142" along normal blind 5 from surface at -1 bodies 3
sketch "Sketch143" plane through (0, 0, 0) normal (0, 0, 1) x (1, 0, 0)
  line L0 (-83.75, 28.75) -> (-97.25, 28.75)
  line L1 (-97.25, 28.75) -> (-97.25, 16.25)
  line L2 (-97.25, 16.25) -> (-83.75, 16.25)
  line L3 (-83.75, 16.25) -> (-83.75, 28.75)
extrude "Extrude143" cut sketch "Sketch143" along normal blind 5 from surface at -1 bodies 3
sketch "Sketch144" plane through (0, 0, 0) normal (0, 0, 1) x (1, 0, 0)
  line L0 (-69.75, 28.75) -> (-83.25, 28.75)
  line L1 (-83.25, 28.75) -> (-83.25, 16.25)
  line L2 (-83.25, 16.25) -> (-69.75, 16.25)
  line L3 (-69.75, 16.25) -> (-69.75, 28.75)
extrude "Extrude144" cut sketch "Sketch144" along normal blind 5 from surface at -1 bodies 3
sketch "Sketch145" plane through (0, 0, 0) normal (0, 0, 1) x (1, 0, 0)
  line L0 (-55.75, 28.75) -> (-69.25, 28.75)
  line L1 (-69.25, 28.75) -> (-69.25, 16.25)
  line L2 (-69.25, 16.25) -> (-55.75, 16.25)
  line L3 (-55.75, 16.25) -> (-55.75, 28.75)
extrude "Extrude145" cut sketch "Sketch145" along normal blind 5 from surface at -1 bodies 3
sketch "Sketch146" plane through (0, 0, 0) normal (0, 0, 1) x (1, 0, 0)
  line L0 (-41.75, 28.75) -> (-55.25, 28.75)
  line L1 (-55.25, 28.75) -> (-55.25, 16.25)
  line L2 (-55.25, 16.25) -> (-41.75, 16.25)
  line L3 (-41.75, 16.25) -> (-41.75, 28.75)
extrude "Extrude146" cut sketch "Sketch146" along normal blind 5 from surface at -1 bodies 3
sketch "Sketch147" plane through (0, 0, 0) normal (0, 0, 1) x (1, 0, 0)
  line L0 (-27.75, 28.75) -> (-41.25, 28.75)
  line L1 (-41.25, 28.75) -> (-41.25, 16.25)
  line L2 (-41.25, 16.25) -> (-27.75, 16.25)
  line L3 (-27.75, 16.25) -> (-27.75, 28.75)
extrude "Extrude147" cut sketch "Sketch147" along normal blind 5 from surface at -1 bodies 3
sketch "Sketch148" plane through (0, 0, 0) normal (0, 0, 1) x (1, 0, 0)
  circle A0 centre (-112, 42) radius 4.5
extrude "Extrude148" cut sketch "Sketch148" along normal blind 5 from surface at -1 bodies 3
sketch "Sketch149" plane through (0, 0, 0) normal (0, 0, 1) x (1, 0, 0)
  line L0 (105.4, 21.2) -> (36.6, 21.2)
  line L1 (36.6, 21.2) -> (36.6, 9.7)
  line L2 (36.6, 9.7) -> (105.4, 9.7)
  line L3 (105.4, 9.7) -> (105.4, 21.2)
extrude "Extrude149" cut sketch "Sketch149" along normal blind 5 from surface at -1 bodies 3
sketch "Sketch150" plane through (0, 0, 0) normal (0, 0, 1) x (1, 0, 0)
  line L0 (1.5, 31) -> (-17.5, 31)
  line L1 (-17.5, 31) -> (-17.5, 18)
  line L2 (-17.5, 18) -> (1.5, 18)
  line L3 (1.5, 18) -> (1.5, 31)
extrude "Extrude150" cut sketch "Sketch150" along normal blind 5 from surface at -1 bodies 3
sketch "Sketch151" plane through (0, 0, 0) normal (0, 0, 1) x (1, 0, 0)
  circle A0 centre (-3, 14.5) radius 3.5
extrude "Extrude151" cut sketch "Sketch151" along normal blind 5 from surface at -1 bodies 3
sketch "Sketch152" plane through (0, 0, 0) normal (0, 0, 1) x (1, 0, 0)
  circle A0 centre (10, 14.5) radius 5
extrude "Extrude152" cut sketch "Sketch152" along normal blind 5 from surface at -1 bodies 3
sketch "Sketch153" plane through (0, 0, 0) normal (0, 0, 1) x (1, 0, 0)
  line L0 (-18.5, 6) -> (-136.7, 6)
  line L1 (-136.7, 6) -> (-136.7, 4)
  line L2 (-136.7, 4) -> (-18.5, 4)
  line L3 (-18.5, 4) -> (-18.5, 6)
extrude "Extrude153" add sketch "Sketch153" along normal blind 10 from surface at -10 bodies 3
sketch "Sketch154" plane through (0, 0, 0) normal (0, 0, 1) x (1, 0, 0)
  line L0 (-18.5, 38) -> (-136.7, 38)
  line L1 (-136.7, 38) -> (-136.7, 36)
  line L2 (-136.7, 36) -> (-18.5, 36)
  line L3 (-18.5, 36) -> (-18.5, 38)
extrude "Extrude154" add sketch "Sketch154" along normal blind 10 from surface at -10 bodies 3
sketch "Sketch155" plane through (0, 0, 0) normal (0, 0, 1) x (1, 0, 0)
  line L0 (-135.5, 36) -> (-136.7, 36)
  line L1 (-136.7, 36) -> (-136.7, 6)
  line L2 (-136.7, 6) -> (-135.5, 6)
  line L3 (-135.5, 6) -> (-135.5, 36)
extrude "Extrude155" add sketch "Sketch155" along normal blind 10 from surface at -10 bodies 3
sketch "Sketch156" plane through (0, 0, 0) normal (0, 0, 1) x (1, 0, 0)
  line L0 (-18.5, 36) -> (-20.5, 36)
  line L1 (-20.5, 36) -> (-20.5, 6)
  line L2 (-20.5, 6) -> (-18.5, 6)
  line L3 (-18.5, 6) -> (-18.5, 36)
extrude "Extrude156" add sketch "Sketch156" along normal blind 10 from surface at -10 bodies 3
sketch "Sketch157" plane through (0, 0, 0) normal (0, 0, 1) x (1, 0, 0)
  line L0 (114.5, 6) -> (27.5, 6)
  line L1 (27.5, 6) -> (27.5, 4)
  line L2 (27.5, 4) -> (114.5, 4)
  line L3 (114.5, 4) -> (114.5, 6)
extrude "Extrude157" add sketch "Sketch157" along normal blind 10 from surface at -10 bodies 3
sketch "Sketch158" plane through (0, 0, 0) normal (0, 0, 1) x (1, 0, 0)
  line L0 (114.5, 32) -> (27.5, 32)
  line L1 (27.5, 32) -> (27.5, 30)
  line L2 (27.5, 30) -> (114.5, 30)
  line L3 (114.5, 30) -> (114.5, 32)
extrude "Extrude158" add sketch "Sketch158" along normal blind 10 from surface at -10 bodies 3
sketch "Sketch159" plane through (0, 0, 0) normal (0, 0, 1) x (1, 0, 0)
  line L0 (29.5, 30) -> (27.5, 30)
  line L1 (27.5, 30) -> (27.5, 6)
  line L2 (27.5, 6) -> (29.5, 6)
  line L3 (29.5, 6) -> (29.5, 30)
extrude "Extrude159" add sketch "Sketch159" along normal blind 10 from surface at -10 bodies 3
sketch "Sketch160" plane through (0, 0, 0) normal (0, 0, 1) x (1, 0, 0)
  line L0 (114.5, 30) -> (112.5, 30)
  line L1 (112.5, 30) -> (112.5, 6)
  line L2 (112.5, 6) -> (114.5, 6)
  line L3 (114.5, 6) -> (114.5, 30)
extrude "Extrude160" add sketch "Sketch160" along normal blind 10 from surface at -10 bodies 3
sketch "Sketch161" plane through (0, 0, 0) normal (0, 0, 1) x (1, 0, 0)
  line L0 (-125, 80) -> (-135, 80)
  line L1 (-135, 80) -> (-135, 76)
  line L2 (-135, 76) -> (-125, 76)
  line L3 (-125, 76) -> (-125, 80)
extrude "Extrude161" add sketch "Sketch161" along normal blind 3 bodies 3
sketch "Sketch162" plane through (0, 0, 0) normal (0, 0, 1) x (1, 0, 0)
  line L0 (-35, 80) -> (-45, 80)
  line L1 (-45, 80) -> (-45, 76)
  line L2 (-45, 76) -> (-35, 76)
  line L3 (-35, 76) -> (-35, 80)
extrude "Extrude162" add sketch "Sketch162" along normal blind 3 bodies 3
sketch "Sketch163" plane through (0, 0, 0) normal (0, 0, 1) x (1, 0, 0)
  line L0 (45, 80) -> (35, 80)
  line L1 (35, 80) -> (35, 76)
  line L2 (35, 76) -> (45, 76)
  line L3 (45, 76) -> (45, 80)
extrude "Extrude163" add sketch "Sketch163" along normal blind 3 bodies 3
sketch "Sketch164" plane through (0, 0, 0) normal (0, 0, 1) x (1, 0, 0)
  line L0 (135, 80) -> (125, 80)
  line L1 (125, 80) -> (125, 76)
  line L2 (125, 76) -> (135, 76)
  line L3 (135, 76) -> (135, 80)
extrude "Extrude164" add sketch "Sketch164" along normal blind 3 bodies 3
sketch "Sketch165" plane through (0, 0, 0) normal (0, 0, 1) x (1, 0, 0)
  circle A0 centre (-120, 72) radius 1.75
extrude "Extrude165" cut sketch "Sketch165" along normal blind 5 from surface at -1 bodies 3
sketch "Sketch166" plane through (0, 0, 0) normal (0, 0, 1) x (1, 0, 0)
  circle A0 centre (-120, 72) radius 3.25
extrude "Extrude166" cut sketch "Sketch166" along normal blind 3 from surface at 0.8 bodies 3
sketch "Sketch167" plane through (0, 0, 0) normal (0, 0, 1) x (1, 0, 0)
  circle A0 centre (-40, 72) radius 1.75
extrude "Extrude167" cut sketch "Sketch167" along normal blind 5 from surface at -1 bodies 3
sketch "Sketch168" plane through (0, 0, 0) normal (0, 0, 1) x (1, 0, 0)
  circle A0 centre (-40, 72) radius 3.25
extrude "Extrude168" cut sketch "Sketch168" along normal blind 3 from surface at 0.8 bodies 3
sketch "Sketch169" plane through (0, 0, 0) normal (0, 0, 1) x (1, 0, 0)
  circle A0 centre (40, 72) radius 1.75
extrude "Extrude169" cut sketch "Sketch169" along normal blind 5 from surface at -1 bodies 3
sketch "Sketch170" plane through (0, 0, 0) normal (0, 0, 1) x (1, 0, 0)
  circle A0 centre (40, 72) radius 3.25
extrude "Extrude170" cut sketch "Sketch170" along normal blind 3 from surface at 0.8 bodies 3
sketch "Sketch171" plane through (0, 0, 0) normal (0, 0, 1) x (1, 0, 0)
  circle A0 centre (120, 72) radius 1.75
extrude "Extrude171" cut sketch "Sketch171" along normal blind 5 from surface at -1 bodies 3
sketch "Sketch172" plane through (0, 0, 0) normal (0, 0, 1) x (1, 0, 0)
  circle A0 centre (120, 72) radius 3.25
extrude "Extrude172" cut sketch "Sketch172" along normal blind 3 from surface at 0.8 bodies 3
sketch "Sketch173" plane through (0, 0, 0) normal (0, 0, 1) x (1, 0, 0)
  circle A0 centre (-132, 44) radius 1.75
extrude "Extrude173" cut sketch "Sketch173" along normal blind 5 from surface at -1 bodies 3
sketch "Sketch174" plane through (0, 0, 0) normal (0, 0, 1) x (1, 0, 0)
  circle A0 centre (-132, 44) radius 3.25
extrude "Extrude174" cut sketch "Sketch174" along normal blind 3 from surface at 0.8 bodies 3
sketch "Sketch175" plane through (0, 0, 0) normal (0, 0, 1) x (1, 0, 0)
  circle A0 centre (132, 44) radius 1.75
extrude "Extrude175" cut sketch "Sketch175" along normal blind 5 from surface at -1 bodies 3
sketch "Sketch176" plane through (0, 0, 0) normal (0, 0, 1) x (1, 0, 0)
  circle A0 centre (132, 44) radius 3.25
extrude "Extrude176" cut sketch "Sketch176" along normal blind 3 from surface at 0.8 bodies 3
sketch "Sketch177" plane through (0, 0, 0) normal (0, 0, 1) x (1, 0, 0)
  line L0 (140, 3) -> (-140, 3)
  line L1 (-140, 3) -> (-140, 0)
  line L2 (-140, 0) -> (140, 0)
  line L3 (140, 0) -> (140, 3)
extrude "Extrude177" add sketch "Sketch177" along normal blind 65 from surface at 3 bodies 3
sketch "Sketch178" plane through (0, 0, 0) normal (0, 0, 1) x (1, 0, 0)
  line L0 (-131, 8) -> (-135, 8)
  line L1 (-135, 8) -> (-135, 3)
  line L2 (-135, 3) -> (-131, 3)
  line L3 (-131, 3) -> (-131, 8)
extrude "Extrude178" add sketch "Sketch178" along normal blind 62 from surface at 3 bodies 3
sketch "Sketch179" plane through (0, 0, 0) normal (0, 0, 1) x (1, 0, 0)
  line L0 (135, 8) -> (131, 8)
  line L1 (131, 8) -> (131, 3)
  line L2 (131, 3) -> (135, 3)
  line L3 (135, 3) -> (135, 8)